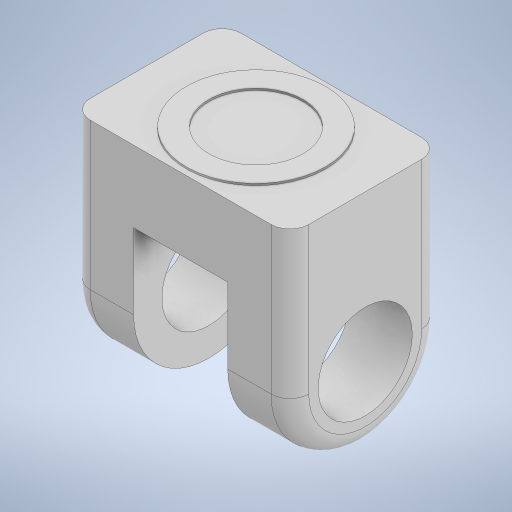
# Autodesk Inventor part: part4
Saved by Autodesk Inventor 2024 (Build 280153000, 153)
## iProperties
Created: 2023-08-22
Part Number: part4
Material: Generic
Document SubType Name: Modeling
Designer: admins
Density: 1 g/cm^3
Appearance: Default
Author: admins
Autodesk Inventor part; units mm, degrees
ref_plane "YZ Plane" through (0, 0, 0) normal (1, 0, 0) x (0, 1, 0)
ref_plane "XZ Plane" through (0, 0, 0) normal (0, 1, 0) x (-1, 0, 0)
ref_plane "XY Plane" through (0, 0, 0) normal (0, 0, 1) x (1, 0, 0)
sketch "Sketch1" plane through (0, 0, 0) normal (0, 1, 0) x (-1, 0, 0)
  line L0 (12.6289, 26.2657) -> (-103.3711, 26.2657)
  line L1 (-103.3711, 26.2657) -> (-103.3711, -53.7343)
  line L2 (-103.3711, -53.7343) -> (12.6289, -53.7343)
  line L3 (12.6289, -53.7343) -> (12.6289, 26.2657)
  point P0 (0, 0)
  dimension "d0" = 116
  dimension "d1" = 80
  constraints: 8 end point, 2 parallel, 1 horizontal, 1 perpendicular
  measures "d0" distance of L2.end L1.end
  measures "d1" distance of L1.end L0.end
extrude "Extrusion1" add sketch "Sketch1" along normal blind 118
sketch "Sketch2" plane through (0, 118, 0) normal (0, 1, 0) x (1, 0, 0)
  circle A0 centre (45.3711, 13.7343) radius 37
  circle A1 centre (45.3711, 13.7343) radius 25
  point P0 (0, 0)
  point P1 (-12.6289, -26.2657)
  dimension "d5" = 74
  dimension "d6" = 50
  constraints: 2 centre point, 1 coincident
  measures "d5" diameter of A0
  measures "d6" diameter of A1
extrude "Extrusion2" add sketch "Sketch2" along normal blind 1
sketch "Sketch3" plane through (103.3711, 0, -53.7343) normal (0, 0, -1) x (-1, 0, 0)
  line L0 (0, 0) -> (116, 0) projected
  line L1 (0, 0) -> (33, 0)
  line L2 (33, 0) -> (83, 0)
  line L3 (83, 0) -> (83, 80)
  line L4 (83, 80) -> (33, 80)
  line L5 (33, 80) -> (33, 0)
  point P0 (103.3711, 0)
  dimension "d9" = 33
  dimension "d10" = 50
  dimension "d11" = 80
  constraints: 10 end point, 2 parallel, 1 horizontal, 1 perpendicular, 1 point on line
  measures "d9" distance of L0.start L1.end
  measures "d10" distance of L4.end L3.end
  measures "d11" distance of L3.end L2.end
extrude "Extrusion3" cut sketch "Sketch3" against normal blind 200
sketch "Sketch4" plane through (-12.6289, 0, -53.7343) normal (-1, 0, 0) x (0, 0, 1)
  circle A0 centre (40, 40) radius 40
  line L0 (0, 0) -> (80, 0) projected
  line L1 (0, 0) -> (0, 118) projected
  circle A1 centre (40, 40) radius 25
  line L2 (0, 0) -> (0, 118) projected
  line L3 (0, 118) -> (80, 118)
  line L4 (80, 118) -> (80, 0)
  line L5 (80, 0) -> (0, 0)
  line L6 (0, 0) -> (0, 118)
  point P0 (53.7343, 0)
  point P1 (0, 40)
  point P2 (40, 0)
  point P3 (80, 40)
  dimension "d14" = 80
  dimension "d15" = 50
  constraints: 8 end point, 2 centre point, 2 parallel, 2 tangent, 1 coincident, 1 horizontal, 1 perpendicular
  measures "d14" diameter of A0
  measures "d15" diameter of A1
extrude "Extrusion4" cut sketch "Sketch4" against normal blind 200 contours A1
extrude "Extrusion5" cut sketch "Sketch4" against normal blind 200 contours A0 L0 L1
extrude "Extrusion6" cut sketch "Sketch4" against normal blind 200 contours L4 L0 A0
fillet "Fillet1" radius 10 6 edges at (-12.6289, 0, -13.7343) (-12.6289, 79, -53.7343) (-12.6289, 79, 26.2657) (103.3711, 0, -13.7343) (103.3711, 79, -53.7343) (103.3711, 79, 26.2657)
body "Solid1"
